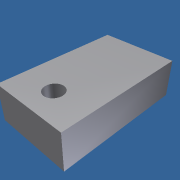
# Autodesk Inventor part: Acrylic_5.8_cameraMount
Saved by Autodesk Inventor 2012 (Build 160160000, 160)
## iProperties
Created: 2014-03-30
Part Number: Acrylic_5.8_cameraMount
Material: Default
Document SubType Name: Modeling
Designer: Admin
Density: 1 g/cm^3
Author: Admin
Autodesk Inventor part; units mm, degrees
ref_plane "YZ Plane" through (0, 0, 0) normal (1, 0, 0) x (0, 1, 0)
ref_plane "XZ Plane" through (0, 0, 0) normal (0, 1, 0) x (-1, 0, 0)
ref_plane "XY Plane" through (0, 0, 0) normal (0, 0, 1) x (1, 0, 0)
sketch "Sketch1" plane through (0, 0, 0) normal (0, 0, 1) x (1, 0, 0)
  line L0 (-8.4, 0) -> (8.4, 0) projected
  line L1 (0, -4) -> (0, 24) projected
  line L2 (-6, 0) -> (6, 0)
  line L3 (6, 0) -> (6, 20)
  line L4 (6, 20) -> (-6, 20)
  line L5 (-6, 20) -> (-6, 0)
  circle A0 centre (0, 4) radius 1.5
  point P0 (0, 0)
  dimension "d0" = 12
  dimension "d1" = 6
  dimension "d2" = 20
  dimension "d3" = 3
  dimension "d4" = 4
  constraints: 8 end point, 2 parallel, 2 point on line, 1 centre point, 1 horizontal, 1 perpendicular
  measures "d0" distance of L3.end L4.end
  measures "d1" distance between parallel lines of L1 L5
  measures "d2" distance of L4.end L2.start
  measures "d3" diameter of A0
  measures "d4" distance from line of L0 A0.centre
extrude "Extrusion1" add sketch "Sketch1" along normal blind 5.8 contours L5 L4 L1 A0 L0 | L1 A0 L4 L3 L0
equation "\"d1\" = 0.5 * d0"
body "Solid1"
